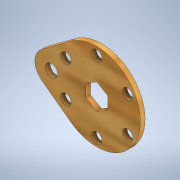
# Autodesk Inventor part: GenevaDrive2
Saved by Autodesk Inventor 2020.1 (Build 241239000, 239)
## iProperties
Created: 2019-11-06
Part Number: GenevaDrive2
Material: Plywood, Finish
Document SubType Name: Modeling
Designer: Paul Lefeuvre
Density: 0.552 g/cm^3
Appearance: Plywood - New
Author: Paul Lefeuvre
Autodesk Inventor part; units mm, degrees
ref_plane "YZ Plane" through (0, 0, 0) normal (1, 0, 0) x (0, 1, 0)
ref_plane "XZ Plane" through (0, 0, 0) normal (0, 1, 0) x (-1, 0, 0)
ref_plane "XY Plane" through (0, 0, 0) normal (0, 0, 1) x (1, 0, 0)
sketch "Sketch1" plane through (0, 0, 0) normal (0, 0, 1) x (1, 0, 0)
  circle A0 centre (0, 0) radius 36.041 construction
  circle A1 centre (-28.541, 0) radius 7.5 construction
  circle A2 centre (0, 0) radius 22.5 construction
  circle A3 centre (0, 22.5) radius 3.3
  circle A4 centre (0, 0) radius 39.041 construction
  arc A5 (-34.7952, 8.4342) -> (-34.7952, -8.4342) centre (-28.541, 0) ccw
  line L0 (-34.7952, 8.4342) -> (-16.3799, 22.0895)
  line L1 (-34.7952, -8.4342) -> (-16.3799, -22.0895)
  line L2 (0, 0) -> (-50.0981, 0) construction
  arc A6 (-16.3799, -22.0895) -> (-16.3799, 22.0895) centre (0, 0) ccw
  circle A7 centre (-19.4856, 11.25) radius 3.3
  circle A8 centre (-19.4856, -11.25) radius 3.3
  circle A9 centre (0, -22.5) radius 3.3
  circle A10 centre (19.4856, -11.25) radius 3.3
  circle A11 centre (19.4856, 11.25) radius 3.3
  line L3 (0, 7.3323) -> (6.35, 3.6662) construction
  line L4 (6.35, 3.6662) -> (6.35, -3.6662) construction
  line L5 (6.35, -3.6662) -> (0, -7.3323) construction
  line L6 (0, -7.3323) -> (-6.35, -3.6662) construction
  line L7 (-6.35, -3.6662) -> (-6.35, 3.6662) construction
  line L8 (-6.35, 3.6662) -> (0, 7.3323) construction
  line L9 (6.95, 4.0126) -> (0, 8.0252)
  line L10 (0, 8.0252) -> (-6.95, 4.0126)
  line L11 (-6.95, 4.0126) -> (-6.95, -4.0126)
  line L12 (-6.95, -4.0126) -> (0, -8.0252)
  line L13 (0, -8.0252) -> (6.95, -4.0126)
  line L14 (6.95, -4.0126) -> (6.95, 4.0126)
  circle A12 centre (-28.541, 0) radius 3.91
  dimension "d17" = 45
  dimension "d2" = 72.082
  dimension "d3" = 15
  dimension "d5" = 6.6
  dimension "d6" = 3
  dimension "d7" = 360
  dimension "d8" = 12.7
  dimension "d9" = 0.6
  dimension "d11" = 7.82
  dimension "d18" = 5
  constraints: 30 end point, 12 centre point, 6 coincident, 6 tangent, 4 point on circle, 1 horizontal, 1 point on line, 1 vertical alignment, 34 other
  measures "d2" diameter of A0
  measures "d3" diameter of A1
  measures "d5" diameter of A3
  measures "d6" radial gap between concentric circles of A4 A0
  measures "d8" distance of L3.end L7.end
  measures "d9" distance between parallel lines of L3 L9
  measures "d11" diameter of A12
extrude "Extrusion1" add sketch "Sketch1" along normal blind 3
body "Solid1"
